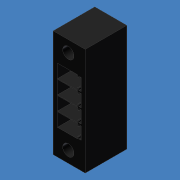
# Autodesk Inventor part: cRIO-FRC Power Connector
Saved by Autodesk Inventor 2011 (Build 150239000, 239)
## iProperties
Category: FRC Parts
Manager: Ed Sparks
Company: FirstCadLibrary
Shininess: 64.0
Length Units: 11272
Angle Units: 11279
Time Units: 11290
Mass Units: 11286
Length Display Precision: 3
Angle Display Precision: 2
Compacted: True
Part Number: cRIO-FRC Power Connector
Document SubType Name: Modeling
Created: 2008-12-13
Designer: Ed Sparks
Project: FIRST
Catalog Web Link: www.firstcadlibrary.com
Engineer: Ed Sparks
Material: ABS Plastic
Density: 1 g/cm^3
Density: 0.0
Volumn: 0.0
Area: 0.0
PropertySet Name: Model Information
Control State: 0
Master: False
Checked Out: False
Author: Ed Sparks
Keywords: FIRST
Autodesk Inventor part; units mm, degrees
ref_plane "YZ Plane" through (0, 0, 0) normal (1, 0, 0) x (0, 1, 0)
ref_plane "XZ Plane" through (0, 0, 0) normal (0, 1, 0) x (-1, 0, 0)
ref_plane "XY Plane" through (0, 0, 0) normal (0, 0, 1) x (1, 0, 0)
sketch "Sketch1" plane through (0, 0, 0) normal (0, 0, 1) x (1, 0, 0)
  line L0 (-3.6195, 12.1158) -> (3.6195, 12.1158)
  line L1 (3.6195, 12.1158) -> (3.6195, -12.1158)
  line L2 (3.6195, -12.1158) -> (-3.6195, -12.1158)
  line L3 (-3.6195, -12.1158) -> (-3.6195, 12.1158)
  line L4 (0, 0) -> (0, 12.1158) construction
  line L5 (0, 0) -> (0, -12.1158) construction
  line L6 (0, 0) -> (-3.6195, 0) construction
  line L7 (0, 0) -> (3.6195, 0) construction
  dimension "d0" = 7.239
  dimension "d1" = 24.2316
  constraints: 16 end point, 4 midpoint, 2 collinear, 2 parallel, 1 horizontal, 1 perpendicular, 1 other
  measures "d0" distance of L0.start L0.end
  measures "d1" distance of L2.end L0.start
extrude "Extrusion1" add sketch "Sketch1" along normal mid plane 9.398
sketch "Sketch2" plane through (0, 0, 4.699) normal (0, 0, 1) x (1, 0, 0)
  line L0 (3.6195, 12.1158) -> (3.6195, -12.1158) projected
  line L1 (-3.6195, -12.1158) -> (-3.6195, 12.1158) projected
  line L2 (-3.6195, 0) -> (3.6195, 0) construction
  point P0 (-0.1905, 9.525)
  dimension "d4" = 9.525
  dimension "d22" = 3.429
  constraints: 2 end point, 2 midpoint
  measures "d4" distance from line of point (-0.19, 9.525) L2
  measures "d22" distance from line of L1 point (-0.19, 9.525)
hole "Hole1" at (-0.1905, 9.525, 4.699) direction (0, 0, -1) diameter 2.54 depth 6.35 tip angle 118
mirror "Mirror1" about plane through (0, 0, 0) normal (0, 1, 0) of "Hole1"
sketch "Sketch3" plane through (0, 0, 4.699) normal (0, 0, 1) x (1, 0, 0)
  line L0 (-3.6195, 12.1158) -> (3.6195, 12.1158) projected
  line L1 (3.6195, -12.1158) -> (-3.6195, -12.1158) projected
  line L2 (-2.667, 6.2865) -> (-2.667, 3.2385)
  line L3 (-2.667, 3.2385) -> (1.905, 3.2385)
  line L4 (1.905, 3.2385) -> (1.905, 3.7465)
  line L5 (1.905, 3.7465) -> (2.159, 3.7465)
  line L6 (2.159, 3.7465) -> (2.159, 3.3655)
  line L7 (2.159, 3.3655) -> (2.667, 3.3655)
  line L8 (2.667, 3.3655) -> (2.667, 6.1595)
  line L9 (2.667, 6.1595) -> (2.159, 6.1595)
  line L10 (2.159, 6.1595) -> (2.159, 5.7785)
  line L11 (2.159, 5.7785) -> (1.905, 5.7785)
  line L12 (1.905, 5.7785) -> (1.905, 6.2865)
  line L13 (1.905, 6.2865) -> (-2.667, 6.2865)
  line L14 (-2.667, 4.7625) -> (2.667, 4.7625) construction
  line L15 (0, 12.1158) -> (0, -12.1158) construction
  point P0 (0, 4.7625)
  dimension "d12" = 3.048
  dimension "d13" = 5.334
  dimension "d14" = 4.572
  dimension "d16" = 2.032
  dimension "d17" = 2.794
  dimension "d18" = 0.508
  dimension "d19" = 5.8293
  constraints: 28 end point, 6 horizontal, 6 vertical, 5 equal length, 5 midpoint, 1 point on line
  measures "d12" distance of L2.start L2.end
  measures "d13" distance between parallel lines of L8 L2
  measures "d14" distance of L2.end L3.end
  measures "d16" distance between parallel lines of L5 L11
  measures "d17" distance between parallel lines of L7 L9
  measures "d18" distance of L6.end L7.end
  measures "d19" distance between parallel lines of L0 L13
extrude "Extrusion2" cut sketch "Sketch3" against normal blind 6.35
pattern_linear "Rectangular Pattern1" count 4 spacing 3.175 along (0, -1, 0) of "Extrusion2"
body "Solid1"
